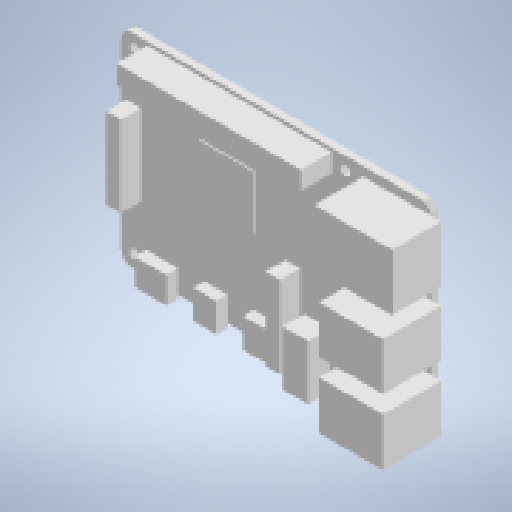
# Autodesk Inventor part: PI 4 B SPACE MODEL
Saved by Autodesk Inventor 2023 (Build 270158000, 158)
## iProperties
Created: 2023-03-17
Part Number: PI 4 B SPACE MODEL
Material: Generic
Document SubType Name: Modeling
Designer: Louis
Density: 1 g/cm^3
Appearance: Default
Author: Louis
Autodesk Inventor part; units mm, degrees
ref_plane "YZ Plane" through (0, 0, 0) normal (1, 0, 0) x (0, 1, 0)
ref_plane "XZ Plane" through (0, 0, 0) normal (0, 1, 0) x (-1, 0, 0)
ref_plane "XY Plane" through (0, 0, 0) normal (0, 0, 1) x (1, 0, 0)
sketch "Sketch1" plane through (0, 0, 0) normal (0, 0, 1) x (1, 0, 0)
  line L0 (-42.5, 28) -> (42.5, 28)
  line L1 (42.5, 28) -> (42.5, -28)
  line L2 (42.5, -28) -> (-42.5, -28)
  line L3 (-42.5, -28) -> (-42.5, 28)
  point P0 (0, 0)
  point P1 (0, 28)
  point P2 (-42.5, 0)
  dimension "d0" = 85
  dimension "d1" = 56
  constraints: 8 end point, 2 midpoint, 2 parallel, 1 horizontal, 1 horizontal alignment, 1 perpendicular, 1 vertical alignment
  measures "d0" distance of L0.start L0.end
  measures "d1" distance of L0.end L1.end
extrude "Extrusion1" add sketch "Sketch1" along normal blind 2
fillet "Fillet1" radius 3 4 edges at (42.5, 28, 1) (42.5, -28, 1) (-42.5, -28, 1) (-42.5, 28, 1)
sketch "Sketch2" plane through (0, 0, 2) normal (0, 0, 1) x (1, 0, 0)
  line L0 (39.5, 28) -> (-39.5, 28) projected
  line L1 (-42.5, 25) -> (-42.5, -25) projected
  line L2 (-39.5, -28) -> (39.5, -28) projected
  point P0 (0, 0)
  point P1 (-39, 24.5)
  point P2 (19, 24.5)
  point P3 (-39, -24.5)
  point P4 (19, -24.5)
  dimension "d5" = 3.5
  dimension "d6" = 3.5
  dimension "d7" = 58
  dimension "d8" = 3.5
  constraints: 2 horizontal alignment, 2 vertical alignment
  measures "d5" distance from line of L0 point (-39, 24.5)
  measures "d6" distance from line of L1 point (-39, 24.5)
  measures "d7" distance of point (19, 24.5) point (-39, 24.5)
  measures "d8" distance from line of L2 point (-39, -24.5)
hole "Hole1" at (-39, 24.5, 2) at (19, 24.5, 2) at (-39, -24.5, 2) at (19, -24.5, 2) direction (0, 0, -1) diameter 2.7 end through all
sketch "Sketch3" plane through (0, 0, 2) normal (0, 0, 1) x (1, 0, 0)
  line L0 (-66.5402, 48.8384) -> (82.1472, 48.8384) construction
  line L1 (82.1472, 48.8384) -> (82.1472, -46.7464) construction
  line L2 (82.1472, -46.7464) -> (-66.5402, -46.7464) construction
  line L3 (-66.5402, -46.7464) -> (-66.5402, 48.8384) construction
  line L4 (27.7, -12.375) -> (45.3, -12.375)
  line L5 (45.3, -12.375) -> (45.3, -25.625)
  line L6 (45.3, -25.625) -> (27.7, -25.625)
  line L7 (27.7, -25.625) -> (27.7, -12.375)
  line L8 (27.7, 5.5) -> (45.3, 5.5)
  line L9 (45.3, 5.5) -> (45.3, -7.5)
  line L10 (45.3, -7.5) -> (27.7, -7.5)
  line L11 (27.7, -7.5) -> (27.7, 5.5)
  line L12 (23.9, 25.5) -> (45.3, 25.5)
  line L13 (45.3, 25.5) -> (45.3, 10)
  line L14 (45.3, 10) -> (23.9, 10)
  line L15 (23.9, 10) -> (23.9, 25.5)
  line L16 (-20.9, 12) -> (-5.9, 12)
  line L17 (-5.9, 12) -> (-5.9, -3)
  line L18 (-5.9, -3) -> (-20.9, -3)
  line L19 (-20.9, -3) -> (-20.9, 12)
  line L20 (-35.75, -21.75) -> (-27, -21.75)
  line L21 (-27, -21.75) -> (-27, -29)
  line L22 (-27, -29) -> (-35.75, -29)
  line L23 (-35.75, -29) -> (-35.75, -21.75)
  line L24 (-13.5, -21.25) -> (-19.75, -21.25)
  line L25 (-19.75, -21.25) -> (-19.75, -29.25)
  line L26 (-19.75, -29.25) -> (-13.5, -29.25)
  line L27 (-13.5, -29.25) -> (-13.5, -21.25)
  line L28 (-6.25, -21.25) -> (0, -21.25)
  line L29 (0, -21.25) -> (0, -29.25)
  line L30 (0, -29.25) -> (-6.25, -29.25)
  line L31 (-6.25, -29.25) -> (-6.25, -21.25)
  line L32 (7.75, -15.25) -> (14.75, -15.25)
  line L33 (14.75, -15.25) -> (14.75, -30.25)
  line L34 (14.75, -30.25) -> (7.75, -30.25)
  line L35 (7.75, -30.25) -> (7.75, -15.25)
  line L36 (2.5, -5) -> (6.5, -5)
  line L37 (6.5, -5) -> (6.5, -27.5)
  line L38 (6.5, -27.5) -> (2.5, -27.5)
  line L39 (2.5, -27.5) -> (2.5, -5)
  line L40 (-37.25, -11) -> (-41.25, -11)
  line L41 (-41.25, -11) -> (-41.25, 11.25)
  line L42 (-41.25, 11.25) -> (-37.25, 11.25)
  line L43 (-37.25, 11.25) -> (-37.25, -11)
  line L44 (-35.5, 27) -> (15.25, 27)
  line L45 (15.25, 27) -> (15.25, 22)
  line L46 (15.25, 22) -> (-35.5, 22)
  line L47 (-35.5, 22) -> (-35.5, 27)
  line L48 (-42.5, 25) -> (-42.5, -25) projected
  line L49 (39.5, 28) -> (-39.5, 28) projected
  line L50 (-39.5, -28) -> (39.5, -28) projected
  line L51 (42.5, -25) -> (42.5, 25) projected
  point P0 (0, 0)
  point P1 (-39.25, 11.25)
  point P2 (45.3, -19)
  point P3 (45.3, -1)
  point P4 (45.3, 17.75)
  dimension "d55" = 7
  dimension "d56" = 50.75
  dimension "d57" = 5
  dimension "d58" = 1
  dimension "d59" = 16.75
  dimension "d60" = 22.25
  dimension "d61" = 4
  dimension "d62" = 1.25
  dimension "d63" = 1
  dimension "d64" = 1.25
  dimension "d65" = 7.25
  dimension "d66" = 8.75
  dimension "d67" = 6.75
  dimension "d68" = 22.75
  dimension "d69" = 6.25
  dimension "d70" = 6.75
  dimension "d71" = 36.25
  dimension "d72" = 6.25
  dimension "d73" = 4
  dimension "d74" = 22.5
  dimension "d75" = 45
  dimension "d76" = 0.5
  dimension "d77" = 7
  dimension "d78" = 2.25
  dimension "d79" = 27.75
  dimension "d80" = 15
  dimension "d81" = 9
  dimension "d82" = 17.6
  dimension "d83" = 13.25
  dimension "d84" = 2.8
  dimension "d85" = 13
  dimension "d86" = 27
  dimension "d87" = 21.4
  dimension "d88" = 15.5
  dimension "d89" = 45.75
  dimension "d90" = 15
  dimension "d91" = 15
  dimension "d92" = 16
  dimension "d93" = 21.6
  constraints: 88 end point, 22 parallel, 11 horizontal, 11 perpendicular, 5 point on line, 4 midpoint, 2 other
  measures "d55" distance from line of L44.start L48
  measures "d56" distance of L44.start L44.end
  measures "d57" distance of L44.end L45.end
  measures "d58" distance between parallel lines of L49 L44
  measures "d59" distance from line of point (-39.25, 11.25) L49
  measures "d60" distance between parallel lines of L40 L42
  measures "d61" distance between parallel lines of L43 L41
  measures "d62" distance between parallel lines of L48 L41
  measures "d63" distance between parallel lines of L50 L22
  measures "d64" distance between parallel lines of L50 L26
  measures "d65" distance of L22.end L20.start
  measures "d66" distance between parallel lines of L21 L23
  measures "d67" distance between parallel lines of L48 L23
  measures "d68" distance between parallel lines of L48 L25
  measures "d69" distance of L24.start L24.end
  measures "d70" distance between parallel lines of L50 L24
  measures "d71" distance between parallel lines of L48 L31
  measures "d72" distance of L28.start L28.end
  measures "d73" distance of L36.start L36.end
  measures "d74" distance of L38.end L36.start
  measures "d75" distance between parallel lines of L48 L39
  measures "d76" distance between parallel lines of L50 L38
  measures "d77" distance of L32.start L32.end
  measures "d78" distance between parallel lines of L50 L34
  measures "d79" distance between parallel lines of L51 L33
  measures "d80" distance of L32.end L33.end
  measures "d81" distance from line of L50 point (45.3, -19)
  measures "d82" distance of L4.start L4.end
  measures "d83" distance of L4.end L5.end
  measures "d84" distance from line of L51 point (45.3, -19)
  measures "d85" distance of L8.end L9.end
  measures "d86" distance from line of L50 point (45.3, -1)
  measures "d87" distance of L12.start L12.end
  measures "d88" distance of L12.end L13.end
  measures "d89" vertical distance of L50.end point (45.3, 17.75)
  measures "d90" distance of L17.end L18.end
  measures "d91" distance of L16.end L17.end
  measures "d92" distance between parallel lines of L49 L16
  measures "d93" distance between parallel lines of L48 L19
extrude "Extrusion2" add sketch "Sketch3" along normal blind 5.5 contours L40 L41 L42 L43
extrude "Extrusion3" add sketch "Sketch3" along normal blind 8.5 contours L44 L45 L46 L47
extrude "Extrusion4" add sketch "Sketch3" along normal blind 2.4 contours L16 L17 L18 L19
extrude "Extrusion5" add sketch "Sketch3" along normal blind 3.2 contours L20 L21 L50 L23 | L50 L21 L22 L23
extrude "Extrusion6" add sketch "Sketch3" along normal blind 3 contours L25 L24 L27 L50 | L50 L27 L26 L25
extrude "Extrusion7" add sketch "Sketch3" along normal blind 3 contours L31 L28 L29 L50 | L50 L29 L30 L31
extrude "Extrusion8" add sketch "Sketch3" along normal blind 5.5 contours L36 L37 L38 L39
extrude "Extrusion9" add sketch "Sketch3" along normal blind 6 contours L35 L32 L33 L50 | L50 L33 L34 L35
extrude "Extrusion10" add sketch "Sketch3" along normal blind 16 contours L4 L5 L6 L7
extrude "Extrusion11" add sketch "Sketch3" along normal blind 16 contours L10 L11 L8 L51 | L51 L8 L9 L10
extrude "Extrusion12" add sketch "Sketch3" along normal blind 13.5 contours L14 L15 L12 L13
sketch "Sketch4" plane through (0, 0, 4.4) normal (0, 0, 1) x (1, 0, 0)
  line L0 (-5.9, -3) -> (-5.9, 12) projected
  line L1 (-20.9, 12) -> (-5.9, 12) projected
  line L2 (-5.9, -3) -> (-20.9, -3)
  line L3 (-20.9, -3) -> (-20.9, 12)
  line L4 (-20.9, 12) -> (-5.9, 12)
  line L5 (-5.9, 12) -> (-5.9, -3)
  point P0 (0, 0)
  constraints: 8 end point, 2 parallel, 1 horizontal, 1 perpendicular
extrude "Extrusion13" cut sketch "Sketch4" against normal blind 2
body "Solid1"
